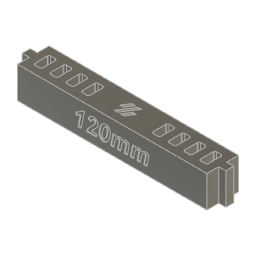
Gantry Support (Autodesk Fusion 360 design; units mm, degrees)
Autodesk Fusion 360 part; units mm, degrees
sketch "Sketch1" plane through (0, 0, 0) normal (0, 0, 1) x (1, 0, 0)
  line L0 (0, 0) -> (120, 0)
  line L1 (120, 20) -> (0, 20)
  line L2 (0, 7.5) -> (-4.5, 7.5)
  line L3 (-4.5, 10) -> (-4.5, 7.5)
  line L4 (0, 12.5) -> (-4.5, 12.5)
  line L5 (-4.5, 12.5) -> (-4.5, 10)
  line L6 (120, 12.5) -> (124.5, 12.5)
  line L7 (124.5, 12.5) -> (124.5, 10)
  line L8 (124.5, 10) -> (124.5, 12.5)
  line L9 (120, 7.5) -> (124.5, 7.5)
  line L10 (124.5, 10) -> (124.5, 7.5)
  line L11 (120, 0) -> (120, 7.5)
  line L12 (120, 12.5) -> (120, 20)
  line L13 (0, 20) -> (0, 12.5)
  line L14 (0, 7.5) -> (0, 0)
  line L15 (5, 14) -> (5, 6)
  line L16 (115, 6) -> (115, 14)
  line L17 (15, 14) -> (15, 6)
  line L18 (10, 6) -> (10, 14)
  line L19 (105, 14) -> (105, 6)
  line L20 (110, 6) -> (110, 14)
  line L21 (95, 14) -> (95, 6)
  line L22 (100, 6) -> (100, 14)
  line L23 (85, 14) -> (85, 6)
  line L24 (90, 6) -> (90, 14)
  line L25 (80, 6) -> (80, 14)
  line L26 (25, 14) -> (25, 6)
  line L27 (20, 6) -> (20, 14)
  line L28 (35, 14) -> (35, 6)
  line L29 (30, 6) -> (30, 14)
  line L30 (40, 6) -> (40, 14)
  line L31 (6, 5) -> (9, 5)
  line L32 (9, 15) -> (6, 15)
  line L33 (19, 15) -> (16, 15)
  line L34 (16, 5) -> (19, 5)
  line L35 (26, 5) -> (29, 5)
  line L36 (29, 15) -> (26, 15)
  line L37 (39, 15) -> (36, 15)
  line L38 (36, 5) -> (39, 5)
  line L39 (111, 5) -> (114, 5)
  line L40 (114, 15) -> (111, 15)
  line L41 (104, 15) -> (101, 15)
  line L42 (101, 5) -> (104, 5)
  line L43 (91, 5) -> (94, 5)
  line L44 (81, 5) -> (84, 5)
  line L45 (94, 15) -> (91, 15)
  line L46 (84, 15) -> (81, 15)
  arc A0 (6, 15) -> (5, 14) centre (6, 14) ccw
  arc A1 (5, 6) -> (6, 5) centre (6, 6) ccw
  arc A2 (9, 5) -> (10, 6) centre (9, 6) ccw
  arc A3 (10, 14) -> (9, 15) centre (9, 14) ccw
  arc A4 (16, 15) -> (15, 14) centre (16, 14) ccw
  arc A5 (15, 6) -> (16, 5) centre (16, 6) ccw
  arc A6 (19, 5) -> (20, 6) centre (19, 6) ccw
  arc A7 (20, 14) -> (19, 15) centre (19, 14) ccw
  arc A8 (26, 15) -> (25, 14) centre (26, 14) ccw
  arc A9 (30, 14) -> (29, 15) centre (29, 14) ccw
  arc A10 (25, 6) -> (26, 5) centre (26, 6) ccw
  arc A11 (29, 5) -> (30, 6) centre (29, 6) ccw
  arc A12 (35, 6) -> (36, 5) centre (36, 6) ccw
  arc A13 (39, 5) -> (40, 6) centre (39, 6) ccw
  arc A14 (40, 14) -> (39, 15) centre (39, 14) ccw
  arc A15 (36, 15) -> (35, 14) centre (36, 14) ccw
  arc A16 (81, 15) -> (80, 14) centre (81, 14) ccw
  arc A17 (80, 6) -> (81, 5) centre (81, 6) ccw
  arc A18 (84, 5) -> (85, 6) centre (84, 6) ccw
  arc A19 (85, 14) -> (84, 15) centre (84, 14) ccw
  arc A20 (91, 15) -> (90, 14) centre (91, 14) ccw
  arc A21 (90, 6) -> (91, 5) centre (91, 6) ccw
  arc A22 (94, 5) -> (95, 6) centre (94, 6) ccw
  arc A23 (95, 14) -> (94, 15) centre (94, 14) ccw
  arc A24 (101, 15) -> (100, 14) centre (101, 14) ccw
  arc A25 (105, 14) -> (104, 15) centre (104, 14) ccw
  arc A26 (104, 5) -> (105, 6) centre (104, 6) ccw
  arc A27 (100, 6) -> (101, 5) centre (101, 6) ccw
  arc A28 (111, 15) -> (110, 14) centre (111, 14) ccw
  arc A29 (110, 6) -> (111, 5) centre (111, 6) ccw
  arc A30 (114, 5) -> (115, 6) centre (114, 6) ccw
  arc A31 (115, 14) -> (114, 15) centre (114, 14) ccw
  line L47 (62.1423, 5.4951) -> (59.9476, 5.4951)
  line L48 (59.9476, 5.4951) -> (62.95, 10.0618)
  line L49 (62.95, 10.0618) -> (65.1447, 10.0618)
  line L50 (65.1447, 10.0618) -> (62.1423, 5.4951)
  line L51 (64.1022, 14.6232) -> (58.0982, 5.4885)
  line L52 (58.0982, 5.4885) -> (55.9034, 5.4885)
  line L53 (55.9034, 5.4885) -> (61.9082, 14.6232)
  line L54 (61.9082, 14.6232) -> (64.1022, 14.6232)
  line L55 (57.8627, 14.6232) -> (60.0574, 14.6232)
  line L56 (60.0574, 14.6232) -> (57.0557, 10.0565)
  line L57 (57.0557, 10.0565) -> (54.861, 10.0565)
  line L58 (54.861, 10.0565) -> (57.8627, 14.6232)
  dimension "d1" = 120
  dimension "d2" = 20
  dimension "d7" = 4.5
  dimension "d10" = 4.5
  dimension "d12" = 1
  constraint horizontal L0
  constraint vertical L11
  constraint horizontal L1
  constraint vertical L13
  constraint coincident L0.start L14.end
  constraint coincident L2.start L13
  constraint perpendicular L2 L13
  constraint perpendicular L4 L13
  constraint coincident L6.start L11
  constraint perpendicular L6 L11
  constraint perpendicular L6 L7
  constraint perpendicular L9 L11
  constraint perpendicular L9 L10
  constraint collinear L11 L12
  constraint collinear L13 L14
  constraint horizontal L40
  constraint vertical L15
  constraint horizontal L31
  constraint vertical L16
  constraint vertical L17
  constraint vertical L18
  constraint vertical L19
  constraint vertical L20
  constraint vertical L21
  constraint vertical L22
  constraint vertical L23
  constraint vertical L24
  constraint vertical L25
  constraint vertical L26
  constraint vertical L27
  constraint vertical L28
  constraint vertical L29
  constraint vertical L30
  constraint collinear L31 L34
  constraint collinear L32 L40
  constraint collinear L33 L40
  constraint collinear L34 L35
  constraint collinear L35 L38
  constraint collinear L36 L40
  constraint collinear L37 L40
  constraint collinear L40 L41
  constraint collinear L41 L45
  constraint collinear L45 L46
  constraint tangent L15 A0
  constraint tangent L32 A0
  constraint tangent L15 A1
  constraint tangent L31 A1
  constraint equal A0 A1
  constraint tangent L31 A2
  constraint tangent L18 A2
  constraint equal A0 A2
  constraint tangent L32 A3
  constraint tangent L18 A3
  constraint equal A0 A3
  constraint tangent L33 A4
  constraint tangent L17 A4
  constraint equal A0 A4
  constraint tangent L17 A5
  constraint tangent L34 A5
  constraint equal A0 A5
  constraint tangent L34 A6
  constraint tangent L27 A6
  constraint equal A0 A6
  constraint tangent L27 A7
  constraint tangent L33 A7
  constraint equal A0 A7
  constraint tangent L36 A8
  constraint tangent L26 A8
  constraint equal A0 A8
  constraint tangent L36 A9
  constraint tangent L29 A9
  constraint equal A0 A9
  constraint tangent L26 A10
  constraint tangent L35 A10
  constraint equal A0 A10
  constraint tangent L35 A11
  constraint tangent L29 A11
  constraint equal A0 A11
  constraint tangent L28 A12
  constraint tangent L38 A12
  constraint equal A0 A12
  constraint tangent L30 A13
  constraint tangent L38 A13
  constraint equal A0 A13
  constraint tangent L30 A14
  constraint tangent L37 A14
  constraint equal A0 A14
  constraint tangent L37 A15
  constraint tangent L28 A15
  constraint equal A0 A15
  constraint tangent L46 A16
  constraint tangent L25 A16
  constraint equal A0 A16
  constraint tangent L25 A17
  constraint tangent L44 A17
  constraint equal A0 A17
  constraint tangent L23 A18
  constraint tangent L44 A18
  constraint equal A0 A18
  constraint tangent L23 A19
  constraint tangent L46 A19
  constraint equal A0 A19
  constraint tangent L45 A20
  constraint tangent L24 A20
  constraint equal A0 A20
  constraint tangent L24 A21
  constraint tangent L43 A21
  constraint equal A0 A21
  constraint tangent L21 A22
  constraint tangent L43 A22
  constraint equal A0 A22
  constraint tangent L21 A23
  constraint tangent L45 A23
  constraint equal A0 A23
  constraint tangent L41 A24
  constraint tangent L22 A24
  constraint equal A0 A24
  constraint tangent L41 A25
  constraint tangent L19 A25
  constraint equal A0 A25
  constraint tangent L19 A26
  constraint tangent L42 A26
  constraint equal A0 A26
  constraint tangent L42 A27
  constraint tangent L22 A27
  constraint equal A0 A27
  constraint tangent L40 A28
  constraint tangent L20 A28
  constraint equal A0 A28
  constraint tangent L20 A29
  constraint tangent L39 A29
  constraint equal A0 A29
  constraint tangent L16 A30
  constraint tangent L39 A30
  constraint equal A0 A30
  constraint tangent L16 A31
  constraint tangent L40 A31
  constraint equal A0 A31
  measures "d1" distance of L0.start L0.end
  measures "d2" distance of L0.start L1.end
  measures "d7" distance of L2.start L2.end
  measures "d10" distance of L6.start L6.end
  measures "d12" radius of A0
extrude "Extrude1" add sketch "Sketch1" along normal blind 20
sketch "Sketch2" plane through (0, 20, 0) normal (0, 1, 0) x (-1, 0, 0)
  line L0 (-120, 0) -> (0, 0)
  line L1 (0, 0) -> (0, 20)
  line L2 (0, 20) -> (-120, 20)
  line L3 (-120, 20) -> (-120, 0)
  line L4 (-119, 1) -> (-1, 1) construction
  line L5 (-1, 1) -> (-1, 19) construction
  line L6 (-1, 19) -> (-119, 19) construction
  line L7 (-119, 19) -> (-119, 1) construction
  dimension "d15" = 10
  text T0 "120mm" font "Arial" height 10 bold italic align centre middle in box 118 x 18 at (-119, 1) x (1, 0) y (0, 1) spacing 1 kerned
extrude "Extrude2" cut sketch "Sketch2" against normal blind 0.5 text T0
sketch "Sketch3" plane through (0, 0, 0) normal (0, -1, 0) x (1, 0, 0)
  line L0 (0, 0) -> (120, 0)
  line L1 (120, 0) -> (120, 20)
  line L2 (120, 20) -> (0, 20)
  line L3 (0, 20) -> (0, 0)
  line L4 (1, 1) -> (119, 1) construction
  line L5 (119, 1) -> (119, 19) construction
  line L6 (119, 19) -> (1, 19) construction
  line L7 (1, 19) -> (1, 1) construction
  dimension "d18" = 10
  text T0 "120mm" font "Arial" height 10 bold italic align centre middle in box 118 x 18 at (1, 1) x (1, 0) y (0, 1) spacing 1 kerned
extrude "Extrude3" cut sketch "Sketch3" against normal blind 0.5 text T0
